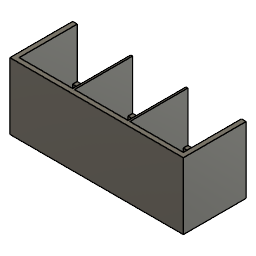
Stepper Housing (Autodesk Fusion 360 design; units mm, degrees)
part number: 2026-02-03-00-25-24-936
Autodesk Fusion 360 part; units mm, degrees
sketch "Sketch1" plane through (0, 0, 0) normal (0, 1, 0) x (1, 0, 0)
  line L0 (-92.1751, -31.3057) -> (92.8249, -31.3057)
  line L1 (92.8249, -31.3057) -> (92.8249, 35.6943)
  line L2 (92.8249, 35.6943) -> (-92.1751, 35.6943)
  line L3 (-92.1751, 35.6943) -> (-92.1751, -31.3057)
  line L4 (87.8249, -26.3057) -> (-87.1751, -26.3057)
  line L5 (-87.1751, -26.3057) -> (-87.1751, 30.6943)
  line L6 (-87.1751, 30.6943) -> (87.8249, 30.6943)
  line L7 (87.8249, 30.6943) -> (87.8249, -26.3057)
  line L8 (30.8249, -26.3057) -> (28.8249, -26.3057)
  line L9 (28.8249, -26.3057) -> (28.8249, 30.6943)
  line L10 (28.8249, 30.6943) -> (30.8249, 30.6943)
  line L11 (30.8249, 30.6943) -> (30.8249, -26.3057)
  line L12 (-30.1751, -26.3057) -> (-28.1751, -26.3057)
  line L13 (-28.1751, -26.3057) -> (-28.1751, 30.6943)
  line L14 (-28.1751, 30.6943) -> (-30.1751, 30.6943)
  line L15 (-30.1751, 30.6943) -> (-30.1751, -26.3057)
  line L16 (-30.1751, 30.6943) -> (-28.1751, 30.6943)
  line L17 (-28.1751, 30.6943) -> (-28.1751, 35.6943)
  line L18 (-28.1751, 35.6943) -> (-30.1751, 35.6943)
  line L19 (-30.1751, 35.6943) -> (-30.1751, 30.6943)
  line L20 (28.8249, 30.6943) -> (30.8249, 30.6943)
  line L21 (30.8249, 30.6943) -> (30.8249, 35.6943)
  line L22 (30.8249, 35.6943) -> (28.8249, 35.6943)
  line L23 (28.8249, 35.6943) -> (28.8249, 30.6943)
  line L24 (87.8249, 30.6943) -> (92.8249, 30.6943)
  line L25 (92.8249, 30.6943) -> (92.8249, 35.6943)
  line L26 (92.8249, 35.6943) -> (87.8249, 35.6943)
  line L27 (87.8249, 35.6943) -> (87.8249, 30.6943)
  line L28 (-87.1751, 30.6943) -> (-92.1751, 30.6943)
  line L29 (-92.1751, 30.6943) -> (-92.1751, 35.6943)
  line L30 (-92.1751, 35.6943) -> (-87.1751, 35.6943)
  line L31 (-87.1751, 35.6943) -> (-87.1751, 30.6943)
  line L32 (87.8249, -26.3057) -> (-87.1751, -26.3057)
  line L33 (-87.1751, -26.3057) -> (-87.1751, -11.3057)
  line L34 (87.8249, -16.2737) -> (87.8249, -26.3057)
  line L35 (87.8249, -26.3057) -> (-87.1751, -26.3057)
  line L36 (-87.1751, -26.3057) -> (-87.1751, -11.3057)
  line L37 (-87.1751, -11.3057) -> (87.8249, -11.3057)
  line L38 (87.8249, -11.3057) -> (87.8249, -26.3057)
  line L39 (92.8249, 2.1943) -> (-92.1751, 2.1943) construction
  dimension "d4" = 57
  dimension "d6" = 5
  dimension "d7" = 5
  dimension "d10" = 57
  dimension "d11" = 57
  dimension "d13" = 2
  dimension "d14" = 2
  dimension "d15" = 5
  dimension "d16" = 5
  dimension "d18" = 2
  dimension "d28" = 2
  dimension "d30" = 5
  dimension "d31" = 15
  dimension "d36" = 57
  constraint horizontal L0
  constraint vertical L1
  constraint horizontal L2
  constraint vertical L3
  constraint horizontal L4
  constraint vertical L5
  constraint horizontal L6
  constraint vertical L7
  constraint horizontal L8
  constraint vertical L9
  constraint horizontal L10
  constraint vertical L11
  constraint coincident L6 L9.end
  constraint coincident L4 L8.start
  constraint horizontal L12
  constraint vertical L13
  constraint horizontal L14
  constraint vertical L15
  constraint coincident L6 L13.end
  constraint coincident L4 L12.start
  constraint horizontal L16
  constraint vertical L17
  constraint horizontal L18
  constraint vertical L19
  constraint coincident L2 L17.end
  constraint horizontal L20
  constraint vertical L21
  constraint horizontal L22
  constraint vertical L23
  constraint horizontal L24
  constraint vertical L25
  constraint horizontal L26
  constraint vertical L27
  constraint horizontal L28
  constraint vertical L29
  constraint horizontal L30
  constraint vertical L31
  constraint horizontal L32
  constraint vertical L33
  constraint vertical L34
  constraint horizontal L35
  constraint vertical L36
  constraint horizontal L37
  constraint vertical L38
  constraint midpoint L1 L39.start
  constraint midpoint L3 L39.end
  measures "d4" distance of L4.start L6.end
  measures "d6" distance of L3 L5
  measures "d7" distance of L0 L4
  measures "d10" distance of L7 L11
  measures "d11" distance of L5 L15
  measures "d13" distance of L13 L15
  measures "d14" distance of L9 L11
  measures "d15" distance of L1 L7
  measures "d16" distance of L2 L6
  measures "d18" distance of L9.end L10.end
  measures "d28" distance of L17 L19
  measures "d30" distance of L6 L22
  measures "d31" distance of L32 L37
  measures "d36" distance of L9 L13
extrude "Extrude1" add sketch "Sketch1" along normal blind 71 contours L0 L1 L3 L4 L5 L7 L8 L12 L24 L28 L32 L33 L34 L35 L36 L38 | L2 L3 L28 L29 L30 L31 | L1 L2 L24 L25 L26 L27 makes body 1
extrude "Extrude2" add sketch "Sketch1" along normal blind 10 contours L5 L6 L15 L37 | L6 L7 L11 L37 | L6 L9 L13 L37 bodies 1 makes body 2 at (9.8249, 0, -16.6943)
extrude "Extrude3" add sketch "Sketch1" along normal blind 71 contours L2 L6 L14 L16 L17 L18 L19 | L6 L13 L14 L15 L16 L37 | L6 L9 L10 L11 L20 L37 | L2 L6 L10 L20 L21 L22 L23 | L4 L12 L13 L15 L32 L35 L37 | L4 L8 L9 L11 L32 L35 L37 bodies 1 2
extrude "Extrude4" add sketch "Sketch1" along normal blind 18 contours L2 L6 L19 L31 | L2 L6 L21 L27 | L2 L6 L17 L23 bodies 1
hole "Hole1" at (82.7852, 10.7785, -35.6943) direction (0, 0, 1) diameter 5 depth 5 tip angle 118 bodies 1
